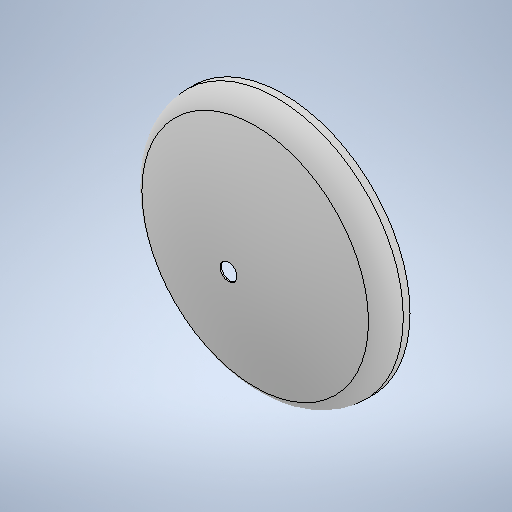
# Autodesk Inventor part: dished head
Saved by Autodesk Inventor 2025 (Build 290162010, 162A)
## iProperties
Created: 2024-12-11
Part Number: dished head
Material: Generic
Document SubType Name: Modeling
Designer: user
Density: 1 g/cm^3
Appearance: Default
Author: user
Autodesk Inventor part; units mm, degrees
ref_plane "YZ Plane" through (0, 0, 0) normal (1, 0, 0) x (0, 1, 0)
ref_plane "XZ Plane" through (0, 0, 0) normal (0, 1, 0) x (-1, 0, 0)
ref_plane "XY Plane" through (0, 0, 0) normal (0, 0, 1) x (1, 0, 0)
sketch "Sketch1" plane through (0, 0, 0) normal (0, 0, 1) x (1, 0, 0)
  line L0 (-671.2707, 588.5845) -> (671.2707, 588.5845) construction
  arc A0 (-671.2707, 588.5845) -> (0, 430) centre (0, 1930) ccw construction
  line L1 (-750, 716.0189) -> (750, 716.0189) construction
  arc A1 (-750, 716.0189) -> (-671.2707, 588.5845) centre (-607.5, 716.0189) ccw construction
  arc A2 (671.2707, 588.5845) -> (750, 716.0189) centre (607.5, 716.0189) ccw
  line L2 (-750, 716.0189) -> (-750, 756.0189)
  line L3 (750, 716.0189) -> (750, 756.0189)
  line L4 (-750, 756.0189) -> (0, 756.0189) construction
  line L5 (0, 756.0189) -> (0, 0)
  arc A3 (0, 430) -> (671.2707, 588.5845) centre (0, 1930) ccw
  line L6 (0, 756.0189) -> (750, 756.0189)
  dimension "d0" = 1500
  dimension "d1" = 142.5
  dimension "d2" = 40
  dimension "d3" = 1500
  dimension "d7_from_floor" = 430
  constraints: 14 end point, 8 point on circle, 4 centre point, 4 tangent, 3 horizontal, 3 vertical, 2 equal length, 1 equal radius, 1 point on line, 1 vertical alignment
  measures "d0" radius of A0
  measures "d1" radius of A1
  measures "d2" distance of L1.start L2.end
  measures "d3" distance of L1.start L1.end
  measures "d7_from_floor" distance of L5.end A0.end
revolve "Revolution1" add sketch "Sketch1" angle 360 about axis through (0, 756.0189, 0) along (0, -1, 0)
shell "Shell1" thickness 8 removed faces 1 at (-43.1672, 756.0189, -310.1274)
sketch "Sketch2" plane through (0, 0, 0) normal (0, 1, 0) x (-1, 0, 0)
  circle A0 centre (0, 0) radius 50
  dimension "d10" = 100
  constraints: 1 centre point, 1 coincident
  measures "d10" diameter of A0
extrude "Extrusion1" cut sketch "Sketch2" along normal through all
equation "\"d0\" = d3"
equation "\"d1\" = 0.095 * d3"
equation "\"d3\" = MAIN_Filter_Diam"
equation "\"d10\" = MAIN_Outer_Tube_Diam"
equation "\"MAIN_Filter_Diam\" = 1500"
equation "\"MAIN_Outer_Tube_Diam\" = 100"
body "Solid1"
